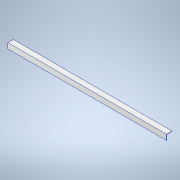
# Autodesk Inventor part: уголок 580
Saved by Autodesk Inventor 2022.4 (Build 264492010, 492A)
## iProperties
Created: 2023-02-20
Part Number: уголок 580
Material: Алюминий 6061
Document SubType Name: Modeling
Designer: artyo
Density: 2.7 g/cm^3
Appearance: Алюминий — плоский
Author: artyo
Autodesk Inventor part; units mm, degrees
ref_plane "YZ Plane" through (0, 0, 0) normal (1, 0, 0) x (0, 1, 0)
ref_plane "XZ Plane" through (0, 0, 0) normal (0, 1, 0) x (-1, 0, 0)
ref_plane "XY Plane" through (0, 0, 0) normal (0, 0, 1) x (1, 0, 0)
sketch "Эскиз1" plane through (0, 0, 0) normal (1, 0, 0) x (0, 1, 0)
  line L0 (-4.5638, 0) -> (-4.5638, 1)
  line L1 (-4.5638, 1) -> (15.4362, 1)
  line L2 (15.4362, 1) -> (15.4362, -19)
  line L3 (15.4362, -19) -> (14.4362, -19)
  line L4 (14.4362, -19) -> (14.4362, 0)
  line L5 (14.4362, 0) -> (-4.5638, 0)
  point P0 (0, 0)
  dimension "d0" = 1
  dimension "d1" = 20
  dimension "d2" = 20
  dimension "d3" = 1
  dimension "d4" = 19
  constraints: 12 end point, 4 perpendicular, 1 vertical
  measures "d0" distance of L0.start L0.end
  measures "d1" distance of L0.end L1.end
  measures "d2" distance of L1.end L2.end
  measures "d3" distance of L2.end L3.end
  measures "d4" distance of L3.end L4.end
extrude "Выдавливание1" add sketch "Эскиз1" along normal blind 580
